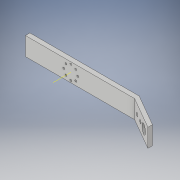
# Autodesk Inventor part: Wheel Arms
Saved by Autodesk Inventor 2019 (Build 230136000, 136)
## iProperties
Created: 2019-10-05
Part Number: Wheel Arms
Material: Generic
Document SubType Name: Modeling
Designer: Delta
Density: 1 g/cm^3
Appearance: Default
Author: Delta
Autodesk Inventor part; units mm, degrees
ref_plane "YZ Plane" through (0, 0, 0) normal (1, 0, 0) x (0, 1, 0)
ref_plane "XZ Plane" through (0, 0, 0) normal (0, 1, 0) x (-1, 0, 0)
ref_plane "XY Plane" through (0, 0, 0) normal (0, 0, 1) x (1, 0, 0)
sketch "Sketch1" plane through (0, 0, 0) normal (0, 0, 1) x (1, 0, 0)
  line L0 (0, 0) -> (152.4, 0)
  line L1 (152.4, 0) -> (152.4, -25.4)
  line L2 (152.4, -25.4) -> (0, -25.4)
  line L3 (0, -25.4) -> (0, 0)
  dimension "d0" = 152.4
  dimension "d1" = 25.4
  constraints: 8 end point, 2 parallel, 1 horizontal, 1 perpendicular
  measures "d0" distance of L1.end L2.end
  measures "d1" distance of L0.end L1.end
extrude "Extrusion1" add sketch "Sketch1" along normal blind 6.35
sketch "Sketch4" plane through (0, 0, 6.35) normal (0, 0, 1) x (1, 0, 0)
  circle A0 centre (63.5, -2.921) radius 1.3589
  circle A1 centre (56.5852, -5.7852) radius 1.3589
  circle A2 centre (53.721, -12.7) radius 1.3589
  circle A3 centre (56.5852, -19.6148) radius 1.3589
  circle A4 centre (63.5, -22.479) radius 1.3589
  circle A5 centre (70.4148, -19.6148) radius 1.3589
  circle A6 centre (73.279, -12.7) radius 1.3589
  circle A7 centre (70.4148, -5.7852) radius 1.3589
  line L0 (0, -25.4) -> (152.4, -25.4) projected
  line L1 (152.4, 0) -> (0, 0) projected
  line L2 (152.4, -25.4) -> (152.4, 0) projected
  point P0 (9.525, 0)
  point P1 (63.5, -12.7)
  point P2 (254, 0)
  point P3 (254, -19.05)
  point P4 (63.5, -12.7)
  point P5 (63.5, -12.7)
  point P6 (63.5, -12.7)
  point P7 (63.5, -12.7)
  point P8 (63.5, -12.7)
  point P9 (63.5, -12.7)
  point P10 (63.5, -12.7)
  point P11 (11.43, 0)
  dimension "d71" = 2.7178
  dimension "d72" = 9.779
  dimension "d73" = 0
  dimension "d76" = 360
  dimension "d85" = 25.4
  dimension "d86" = 12.7
  dimension "d87" = 88.9
  constraints: 8 centre point, 2 coincident, 23 other
  measures "d71" diameter of A0
  measures "d72" distance of point (63.5, -12.7) A0.centre
  measures "d73" horizontal distance of A0.centre point (63.5, -12.7)
  measures "d85" distance between parallel lines of L0 L1
  measures "d86" distance from line of L1 point (63.5, -12.7)
  measures "d87" distance from line of L2 point (63.5, -12.7)
sketch "Sketch9" plane through (152.4, -25.4, 0) normal (0, -1, 0) x (1, 0, 0)
  line L0 (0, 0) -> (0, 6.35) projected
  line L1 (0, 0) -> (43.9941, 25.4)
  line L2 (0, 0) -> (50.8, 0) construction
  line L3 (0, 6.35) -> (43.9941, 31.75)
  line L4 (0, 6.35) -> (50.8, 6.35) construction
  line L5 (43.9941, 31.75) -> (43.9941, 25.4)
  point P0 (-152.4, 0)
  dimension "d53" = 50.8
  dimension "d54" = 30
  dimension "d55" = 50.8
  dimension "d56" = 30
  constraints: 10 end point, 2 equal length, 2 horizontal
  measures "d53" distance of L0.start L1.end
  measures "d54" angle of L2 L1
  measures "d55" distance of L0.end L3.end
  measures "d56" angle of L4 L3
extrude "Extrusion9" add sketch "Sketch9" against normal up to surface (25.4 mm away)
sketch "Sketch10" plane through (196.3941, -25.4, 25.4) normal (0.5, 0, -0.8660254) x (-0.8660254, 0, -0.5)
  line L0 (0, 0) -> (50.8, 0) projected
  line L1 (50.8, 25.4) -> (0, 25.4) projected
  line L2 (0, 0) -> (0, 25.4) projected
  circle A0 centre (38.1, 12.7) radius 2.3368
  circle A1 centre (25.4, 12.7) radius 2.3368
  circle A2 centre (12.7, 12.7) radius 6.35
  point P0 (182.7823, 25.4)
  dimension "d59" = 25.4
  dimension "d60" = 12.7
  dimension "d61" = 12.7
  dimension "d62" = 12.7
  dimension "d63" = 12.7
  dimension "d64" = 25.4
  dimension "d65" = 38.1
  dimension "d66" = 4.6736
  dimension "d67" = 4.6736
  dimension "d68" = 12.7
  constraints: 3 centre point, 3 coincident
  measures "d59" distance between parallel lines of L0 L1
  measures "d60" distance from line of L0 point (38.1, 12.7)
  measures "d61" distance from line of L0 point (25.4, 12.7)
  measures "d62" distance from line of L0 point (12.7, 12.7)
  measures "d63" distance from line of L2 point (12.7, 12.7)
  measures "d64" distance from line of L2 point (25.4, 12.7)
  measures "d65" distance from line of L2 point (38.1, 12.7)
  measures "d66" diameter of A0
  measures "d67" diameter of A1
  measures "d68" diameter of A2
extrude "Extrusion10" cut sketch "Sketch10" against normal through all
hole "Hole1" at (70.4148, -5.7852, 6.35) at (73.279, -12.7, 6.35) at (70.4148, -19.6148, 6.35) at (63.5, -22.479, 6.35) at (56.5852, -19.6148, 6.35) at (53.721, -12.7, 6.35) at (56.5852, -5.7852, 6.35) at (63.5, -2.921, 6.35) direction (0, 0, -1) diameter 2.7178 end through all
equation "\"d86\" = 0.5 * d85"
equation "\"d55\" = d53"
equation "\"d60\" = 0.5 * d59"
equation "\"d61\" = d60"
equation "\"d62\" = d60"
body "Solid1"
